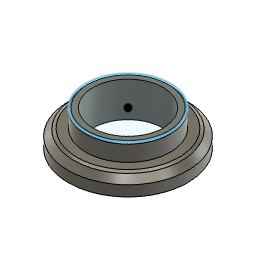
nixie_rohr_mount_24x30 v4 (Autodesk Fusion 360 design; units mm, degrees)
Autodesk Fusion 360 part; units mm, degrees
sketch "Skizze1" plane through (0, 0, 0) normal (0, 1, 0) x (1, 0, 0)
  circle A0 centre (0, 0) radius 10
  line L0 (0, 0) -> (-35, 0)
  circle A1 centre (-35, 0) radius 10
  circle A2 centre (0, 0) radius 12
  circle A3 centre (0, 0) radius 15
  circle A4 centre (-35, 0) radius 12
  circle A5 centre (-35, 0) radius 15
  circle A6 centre (0, 0) radius 17
  circle A7 centre (0, 0) radius 11.75
  dimension "d1" = 20
  dimension "d2" = 35
  dimension "d3" = 20
  dimension "d4" = 24
  dimension "d5" = 30
  dimension "d6" = 24
  dimension "d7" = 30
  dimension "d12" = 34
  dimension "d20" = 23.5
  constraint coincident A0.centre L0.start
  constraint horizontal L0
  constraint coincident L0.end A1.centre
  constraint concentric A0 A2
  constraint concentric A2 A3
  constraint concentric A1 A4
  constraint concentric A4 A5
  constraint concentric A3 A6
  constraint concentric A6 A7
  measures "d1" diameter of A0
  measures "d2" distance of A0.centre L0.end
  measures "d3" diameter of A1
  measures "d4" diameter of A2
  measures "d5" diameter of A3
  measures "d6" diameter of A4
  measures "d7" diameter of A5
  measures "d12" diameter of A6
  measures "d20" diameter of A7
extrude "Extrusion3" add sketch "Skizze1" along normal blind 5 contours A6
chamfer "Fase1" distance 2 angle 45 1 edges at (-15.8496, 5, 6.1475)
extrude "Extrusion4" add sketch "Skizze1" along normal blind 5 contours A3
extrude "Extrusion5" add sketch "Skizze1" along normal blind 10 contours A2 | A7
sketch "Skizze2" plane through (0, 10, 0) normal (0, 1, 0) x (-1, 0, 0)
  circle A0 centre (0, 0) radius 10
  circle A1 centre (0, 0) radius 12
  circle A2 centre (0, 0) radius 12
  circle A3 centre (0, 0) radius 11.75
  constraint coincident A0.centre A1.centre
extrude "Extrusion6" cut sketch "Skizze2" against normal blind 5 contours A1 A2
extrude "Extrusion7" add sketch "Skizze1" along normal blind 9 contours A2
extrude "Extrusion8" add 1 faces at (-11.872, 9, 0.5962) along direction (0, 1, 0) blind 1
chamfer "Fase2" distance 0.5 angle 45 1 edges at (-13.9849, 5, -5.4242)
chamfer "Fase3" distance 0.5 angle 45 1 edges at (-11.1879, 10, 4.3394)
sketch "Skizze3" plane through (0, 10, 0) normal (0, 1, 0) x (-1, 0, 0)
  circle A0 centre (0, 0) radius 10
  circle A1 centre (0, 0) radius 11.5
  circle A2 centre (0, 0) radius 12
  constraint coincident A0.centre A1.centre
